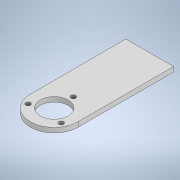
# Autodesk Inventor part: Focuser Base
Saved by Autodesk Inventor 2020.2 (Build 242310000, 310)
## iProperties
Created: 2019-12-22
Part Number: Focuser Base
Material: Generic
Document SubType Name: Modeling
Designer: robst
Density: 1 g/cm^3
Appearance: Default
Author: robst
Autodesk Inventor part; units mm, degrees
ref_plane "YZ Plane" through (0, 0, 0) normal (1, 0, 0) x (0, 1, 0)
ref_plane "XZ Plane" through (0, 0, 0) normal (0, 1, 0) x (-1, 0, 0)
ref_plane "XY Plane" through (0, 0, 0) normal (0, 0, 1) x (1, 0, 0)
sketch "Sketch1" plane through (0, 0, 0) normal (0, 1, 0) x (-1, 0, 0)
  circle A0 centre (0, 0) radius 15.24 construction
  circle A1 centre (0, -15.24) radius 1.905
  circle A2 centre (13.1982, 7.62) radius 1.905
  circle A3 centre (-13.1982, 7.62) radius 1.905
  arc A4 (19.05, 0) -> (-19.05, 0) centre (0, 0) ccw
  line L0 (19.05, 0) -> (19.05, -76.2)
  line L1 (19.05, -76.2) -> (-19.05, -76.2)
  line L2 (-19.05, -76.2) -> (-19.05, 0)
  circle A5 centre (0, 0) radius 11.1125
  point P0 (0, -19.05)
  point P1 (0, 19.05)
  dimension "boltHoleDiameter" = 30.48
  dimension "d1" = 3.81
  dimension "d4" = 360
  dimension "exteriorOfBolts" = 38.1
  dimension "majorLength" = 76.2
  dimension "d12" = 22.225
  constraints: 6 end point, 5 centre point, 4 point on circle, 3 coincident, 1 horizontal, 1 perpendicular, 1 vertical, 1 vertical alignment, 9 other
  measures "d1" diameter of A1
  measures "exteriorOfBolts" diameter of A4
  measures "majorLength" distance of L0.start L0.end
  measures "d12" diameter of A5
extrude "Extrusion2" add sketch "Sketch1" against normal blind 3.81
body "Solid2"
